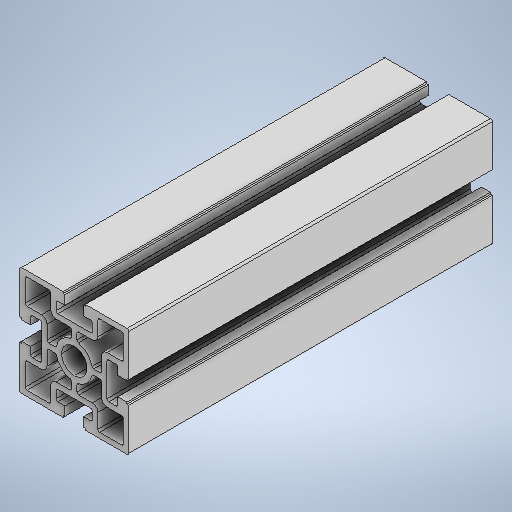
# Autodesk Inventor part: profile_60x60_0001_0001
Saved by Autodesk Inventor 2025.2 (Build 292293000, 293)
## iProperties
Created: 2025-04-05
Part Number: profile_60x60_0001_0001
Material: Generic
Document SubType Name: Modeling
Designer: kenne
Density: 1 g/cm^3
Appearance: Default
Author: kenne
Autodesk Inventor part; units mm, degrees
ref_plane "YZ Plane" through (0, 0, 0) normal (1, 0, 0) x (0, 1, 0)
ref_plane "XZ Plane" through (0, 0, 0) normal (0, 1, 0) x (-1, 0, 0)
ref_plane "XY Plane" through (0, 0, 0) normal (0, 0, 1) x (1, 0, 0)
sketch "profile_Sketch" plane through (0, 0, 0) normal (0, 0, 1) x (1, 0, 0)
  line L0 (-30, 30) -> (30, 30) construction
  line L1 (-30, 30) -> (-30, 5.1) construction
  line L2 (-29, 30) -> (-5.1, 30) construction
  line L3 (-5.1, 30) -> (-5.1, 24) construction
  line L4 (-30, 5.1) -> (-24, 5.1) construction
  circle A0 centre (0, 0) radius 7 construction
  line L5 (0, 0) -> (-30, 30) construction
  line L6 (-27, 27) -> (-13, 27) construction
  line L7 (-13, 27) -> (-13, 13) construction
  line L8 (-13, 13) -> (-27, 13) construction
  line L9 (-27, 13) -> (-27, 27) construction
  line L10 (-24, 5.1) -> (-24, 9)
  line L11 (-23, 10) -> (-19, 10)
  line L12 (-18, 9) -> (-18, 5.1)
  line L13 (-18, 5.1) -> (-18, 0)
  circle A1 centre (0, 0) radius 10 construction
  line L14 (-10.7121, 1.5) -> (-14, 1.5)
  line L15 (-27, 13) -> (-18, 13) construction
  line L16 (-5.1, 24) -> (-9, 24)
  line L17 (-10, 23) -> (-10, 19)
  line L18 (0, 30) -> (0, 10) construction
  line L19 (-9, 18) -> (0, 18)
  line L20 (-1.5, 10.7121) -> (-1.5, 14) construction
  arc A2 (-2.2727, 9.7383) -> (-9.7383, 2.2727) centre (0, 0) ccw
  line L21 (-2.5, 15) -> (-10, 15) construction
  line L22 (-13, 27) -> (-13, 18) construction
  line L23 (-15, 2.5) -> (-15, 10)
  arc A3 (-13, 18) -> (-10, 15) centre (-10, 18) ccw
  arc A4 (-15, 10) -> (-18, 13) centre (-18, 10) ccw
  arc A5 (0, 7) -> (-7, 0) centre (-0.0022, 0.0022) ccw
  line L24 (-7, 0) -> (-18, 0)
  line L25 (0, 18) -> (0, 7)
  arc A6 (-26, 27) -> (-27, 26) centre (-26, 26) ccw
  arc A7 (-13, 26) -> (-14, 27) centre (-14, 26) ccw
  line L26 (-26, 27) -> (-14, 27)
  line L27 (-13, 26) -> (-13, 18)
  arc A8 (-27, 14) -> (-26, 13) centre (-26, 14) ccw
  line L28 (-27, 26) -> (-27, 14)
  line L29 (-26, 13) -> (-18, 13)
  arc A9 (-1.5, 14) -> (-2.5, 15) centre (-2.5, 14) ccw
  arc A10 (-2.2727, 9.7383) -> (-1.5, 10.7121) centre (-2.5, 10.7121) ccw
  line L30 (-10, 15) -> (-2.5, 15)
  line L31 (-1.5, 14) -> (-1.5, 10.7121)
  arc A11 (-10.7121, 1.5) -> (-9.7383, 2.2727) centre (-10.7121, 2.5) ccw
  arc A12 (-15, 2.5) -> (-14, 1.5) centre (-14, 2.5) ccw
  arc A13 (-9, 24) -> (-10, 23) centre (-9, 23) ccw
  arc A14 (-10, 19) -> (-9, 18) centre (-9, 19) ccw
  arc A15 (-18, 9) -> (-19, 10) centre (-19, 9) ccw
  line L32 (-30, 5.1) -> (-29, 5.1) construction
  line L33 (-29, 5.1) -> (-29, 6.1)
  line L34 (-29, 6.1) -> (-30, 6.1)
  line L35 (-30, 6.1) -> (-30, 5.1) construction
  line L36 (-29, 5.1) -> (-24, 5.1)
  line L37 (-30, 6.1) -> (-30, 29)
  arc A16 (-29, 30) -> (-30, 29) centre (-29, 29) ccw
  line L38 (-5.1, 30) -> (-6.1, 30) construction
  line L39 (-6.1, 30) -> (-6.1, 29)
  line L40 (-6.1, 29) -> (-5.1, 29)
  line L41 (-5.1, 29) -> (-5.1, 30) construction
  line L42 (-5.1, 29) -> (-5.1, 24)
  line L43 (-29, 30) -> (-6.1, 30)
  arc A17 (-23, 10) -> (-24, 9) centre (-23, 9) ccw
  point P0 (-24, 10)
  point P1 (-18, 10)
  point P2 (-18, 0)
  point P3 (-9.8869, 1.5)
  point P4 (-15, 1.5)
  point P5 (-10, 24)
  point P6 (-10, 18)
  point P7 (-1.5, 9.8869)
  point P8 (-1.5, 15)
  dimension "d0" = 30
  dimension "width" = 60
  dimension "d3" = 24.9
  dimension "d4" = 5.1
  dimension "expessura" = 6
  dimension "d6" = 6
  dimension "d7" = 14
  dimension "d10" = 3
  dimension "d11" = 14
  dimension "d12" = 3
  dimension "d15" = 6
  dimension "d16" = 3
  dimension "d19" = 3
  dimension "d20" = 6
  dimension "d21" = 1.5
  dimension "d22" = 3
  dimension "d23" = 10
  dimension "d24" = 3
  dimension "d25" = 6.9978
  dimension "d26" = 8.5
  dimension "d27" = 11
  dimension "d30" = 1
  dimension "d31" = 1
  dimension "d32" = 1
  dimension "d33" = 1
  dimension "d34" = 1
  dimension "d35" = 1
  dimension "d37" = 1
  dimension "d38" = 1
  dimension "d39" = 1
  dimension "d40" = 1
  constraints: 88 end point, 39 point on circle, 30 point on line, 27 tangent, 18 centre point, 11 horizontal, 10 vertical, 6 collinear, 6 parallel, 6 perpendicular, 4 equal radius, 4 vertical alignment, 3 equal length, 2 coincident, 2 horizontal alignment, 1 midpoint
  measures "d0" distance from line of point (0, 0) L0
  measures "width" distance of L0.start L0.end
  measures "d3" distance of L0.start L1.end
  measures "d4" distance of L18.start L2.end
  measures "expessura" distance of L2.end L3.end
  measures "d6" distance of L1.end L4.end
  measures "d7" diameter of A0
  measures "d10" distance between parallel lines of L9 L1
  measures "d11" distance between parallel lines of L8 L6
  measures "d12" distance from line of point (-24, 10) L8
  measures "d15" distance of point (-24, 10) point (-18, 10)
  measures "d16" radial gap between concentric circles of A0 A1
  measures "d19" distance from line of point (-10, 24) L7
  measures "d20" distance of point (-10, 24) point (-10, 18)
  measures "d21" distance between parallel lines of L18 L20
  measures "d22" distance from line of L19 point (-1.5, 15)
  measures "d23" radius of A2
  measures "d24" distance between parallel lines of L23 L12
  measures "d25" radius of A5
  measures "d26" distance of point (-15, 1.5) L23.end
  measures "d27" distance of L24.start point (-18, 0)
  measures "d30" radius of A6
  measures "d31" radius of A7
  measures "d32" radius of A8
  measures "d33" radius of A9
  measures "d34" radius of A10
  measures "d35" radius of A11
  measures "d37" distance of L33.end L34.end
  measures "d38" radius of A16
  measures "d39" distance of L38.end L39.end
  measures "d40" radius of A17
extrude "profile_Extrusion" add sketch "profile_Sketch" along normal mid plane 200
mirror "Mirror3" about plane through (0, 0, 0) normal (1, 0, 0) of "profile_Extrusion"
mirror "Mirror4" about plane through (0, 0, 0) normal (0, 1, 0) of "profile_Extrusion", "Mirror3"
equation "\"d6\" = expessura"
body "Solid2"
